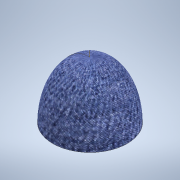
# Autodesk Inventor part: Egg Capsule Top
Saved by Autodesk Inventor 2022 (Build 260153000, 153)
## iProperties
Created: 2022-02-15
Part Number: Egg Capsule Top
Material: Generic
Document SubType Name: Modeling
Designer: Nathan Griffith
Density: 1 g/cm^3
Appearance: Denim - Blue
Author: Nathan Griffith
Autodesk Inventor part; units mm, degrees
ref_plane "YZ Plane" through (0, 0, 0) normal (1, 0, 0) x (0, 1, 0)
ref_plane "XZ Plane" through (0, 0, 0) normal (0, 1, 0) x (-1, 0, 0)
ref_plane "XY Plane" through (0, 0, 0) normal (0, 0, 1) x (1, 0, 0)
sketch "Sketch1" plane through (0, 0, 0) normal (0, 0, 1) x (1, 0, 0)
  line L0 (18.415, -31.115) -> (-18.415, -31.115)
  line L1 (-18.415, -31.115) -> (-18.415, 31.115)
  line L2 (-18.415, 31.115) -> (0, 31.115)
  line L3 (18.415, -31.115) -> (-18.415, 31.115) construction
  line L4 (-18.415, -31.115) -> (18.415, 31.115) construction
  ellipse E0 centre (0, 0) end of major axis (0, 31.115) minor radius 18.415 (0, 31.115) -> (0, -31.115) ccw
  line L5 (0, 31.115) -> (0, -31.115)
  line L6 (-18.415, 0) -> (0, 0)
  line L7 (-18.415, 31.115) -> (18.415, 31.115) construction
  dimension "d0" = 36.83
  dimension "d1" = 62.23
  constraints: 16 end point, 4 midpoint, 3 horizontal, 1 coincident, 1 parallel, 1 perpendicular, 1 vertical, 5 other
  measures "d0" distance of L1.end L4.end
  measures "d1" distance of L0.end L1.end
revolve "Revolution1" add sketch "Sketch1" angle 360 about axis through (0, 31.115, 0) along (0, -1, 0) picked at (-3.6353, 18.7288) contours E0 L5 L6
shell "Shell1" thickness 6.35 outward yes removed faces 1 at (-4.5946, 0, -1.6348)
sketch "Sketch13" plane through (0, 0, 0) normal (0, -1, 0) x (1, 0, 0)
  circle A0 centre (0, 0) radius 18.415 projected
  circle A1 centre (0, 0) radius 24.765 projected
  circle A2 centre (0, 0) radius 21.59
  circle A3 centre (0, 0) radius 22.86
  circle A4 centre (0, 0) radius 20.32
  point P0 (0, 0)
  point P1 (-18.415, 0)
  point P2 (-24.765, 0)
  dimension "d52" = 49.53
  dimension "d53" = 36.83
  dimension "d54" = 43.18
  dimension "d55" = 1.27
  dimension "d56" = 1.27
  dimension "d59" = 45.72
  constraints: 3 centre point, 2 horizontal alignment, 1 coincident
  measures "d54" diameter of A2
  measures "d55" radial gap between concentric circles of A2 A3
  measures "d56" radial gap between concentric circles of A2 A4
  measures "d59" diameter of A3
extrude "Extrusion9" cut sketch "Sketch13" against normal blind 6.35 contours A2 | A3
sketch "Sketch16" plane through (0, 0, 0) normal (1, 0, 0) x (0, 1, 0)
  line L0 (5.334, -22.86) -> (7.366, -22.86)
  line L1 (7.366, -22.86) -> (6.35, -23.9362)
  line L2 (6.35, -23.9362) -> (5.334, -22.86)
  point P0 (0, 0)
  dimension "d70" = 2.032
  constraints: 6 end point, 1 equal length, 1 horizontal, 1 horizontal alignment, 1 midpoint
  measures "d70" distance of L0.start L0.end
sketch3d "3D Sketch1"
  helix H0 starts at (0, 6.35, -22.86) axis through (0, 6.35, 0) along (0, -1, 0) pitch 2.1167 turns 3 hand right
sweep "Sweep1" cut profiles "Sketch16" path "3D Sketch1"
equation "\"d54\" = 0.5 * d52 + 0.5 * d53"
body "Solid1"
